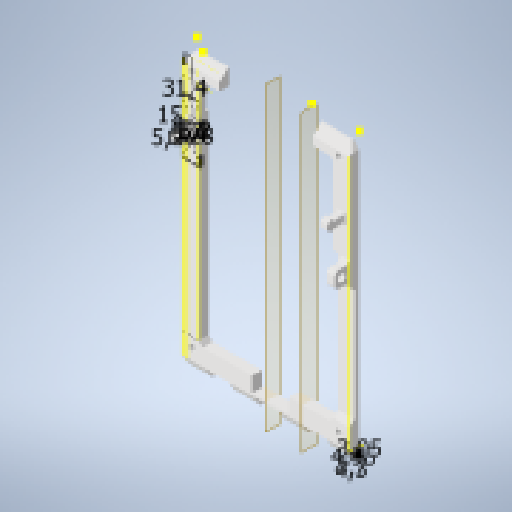
# Autodesk Inventor part: cap
Saved by Autodesk Inventor 2025 (Build 290162000, 162)
## iProperties
Created: 2026-10-31
Part Number: cap
Material: Типовые
Document SubType Name: Modeling
Designer: Leva
Density: 1 g/cm^3
Appearance: По умолчанию
Author: Leva
Autodesk Inventor part; units mm, degrees
ref_plane "YZ Plane" through (0, 0, 0) normal (1, 0, 0) x (0, 1, 0)
ref_plane "XZ Plane" through (0, 0, 0) normal (0, 1, 0) x (-1, 0, 0)
ref_plane "XY Plane" through (0, 0, 0) normal (0, 0, 1) x (1, 0, 0)
sketch "Эскиз1" plane through (0, 0, 0) normal (0, 0, 1) x (1, 0, 0)
  line L0 (72.7181, -132.5726) -> (72.7181, -8.0726) projected
  line L1 (72.7181, -8.0726) -> (69.7181, -5.0726) projected
  line L2 (69.7181, -5.0726) -> (-7.2819, -5.0726) projected
  line L3 (-7.2819, -5.0726) -> (-10.2819, -8.0726) projected
  line L4 (-10.2819, -8.0726) -> (-10.2819, -132.5726) projected
  line L5 (-10.2819, -132.5726) -> (-7.2819, -135.5726) projected
  line L6 (-7.2819, -135.5726) -> (69.7181, -135.5726) projected
  line L7 (69.7181, -135.5726) -> (72.7181, -132.5726) projected
  circle A0 centre (37.8631, -131.3876) radius 0.325 projected
  circle A1 centre (37.8631, -132.6576) radius 0.325 projected
  circle A2 centre (67.7181, -130.5726) radius 1.35 projected
  circle A3 centre (54.6891, -79.8326) radius 1.55 projected
  circle A4 centre (36.5931, -132.6576) radius 0.325 projected
  circle A5 centre (35.3231, -132.6576) radius 0.325 projected
  line L8 (17.4681, -90.7666) -> (44.9681, -90.7666) projected
  arc A6 (11.5241, -84.8226) -> (17.4681, -90.7666) centre (17.4683, -84.8225) ccw projected
  line L9 (11.5241, -57.3226) -> (11.5241, -84.8226) projected
  arc A7 (17.4681, -51.3786) -> (11.5241, -57.3226) centre (17.4683, -57.3227) ccw projected
  line L10 (44.9681, -51.3786) -> (17.4681, -51.3786) projected
  arc A8 (50.9121, -57.3226) -> (44.9681, -51.3786) centre (44.968, -57.3227) ccw projected
  line L11 (50.9121, -84.8226) -> (50.9121, -57.3226) projected
  arc A9 (44.9681, -90.7666) -> (50.9121, -84.8226) centre (44.968, -84.8225) ccw projected
  circle A10 centre (35.3231, -131.3876) radius 0.325 projected
  circle A11 centre (36.5931, -131.3876) radius 0.325 projected
  circle A12 centre (60.4681, -32.7976) radius 0.45 projected
  circle A13 centre (58.4681, -32.7976) radius 0.45 projected
  circle A14 centre (67.7181, -11.5726) radius 1.35 projected
  circle A15 centre (58.4681, -28.2976) radius 0.45 projected
  circle A16 centre (60.4681, -28.2976) radius 0.45 projected
  circle A17 centre (56.4361, -32.7976) radius 0.45 projected
  circle A18 centre (50.9731, -42.2126) radius 1.1 projected
  circle A19 centre (56.4681, -28.2976) radius 0.45 projected
  line L12 (48.1131, -37.9766) -> (14.3131, -37.9766) projected
  line L13 (14.3131, -37.9766) -> (14.3131, -7.4766) projected
  line L14 (14.3131, -7.4766) -> (48.1131, -7.4766) projected
  line L15 (48.1131, -7.4766) -> (48.1131, -37.9766) projected
  circle A20 centre (50.9731, -10.1686) radius 1.1 projected
  circle A21 centre (34.0531, -132.6576) radius 0.325 projected
  circle A22 centre (32.7831, -132.6576) radius 0.325 projected
  circle A23 centre (34.0531, -131.3876) radius 0.325 projected
  circle A24 centre (32.7831, -131.3876) radius 0.325 projected
  circle A25 centre (31.5131, -132.6576) radius 0.325 projected
  circle A26 centre (30.2431, -132.6576) radius 0.325 projected
  circle A27 centre (31.5131, -131.3876) radius 0.325 projected
  circle A28 centre (28.9731, -132.6576) radius 0.325 projected
  circle A29 centre (-5.2819, -130.5726) radius 1.35 projected
  circle A30 centre (30.2431, -131.3876) radius 0.325 projected
  circle A31 centre (28.9731, -131.3876) radius 0.325 projected
  circle A32 centre (34.2431, -122.5726) radius 1.1 projected
  circle A33 centre (34.2431, -97.5726) radius 1.1 projected
  circle A34 centre (31.2891, -47.9156) radius 1.55 projected
  circle A35 centre (11.2431, -96.7726) radius 1.1 projected
  circle A36 centre (7.8891, -79.8326) radius 1.55 projected
  circle A37 centre (11.4731, -42.2126) radius 1.1 projected
  circle A38 centre (-5.2819, -11.5726) radius 1.35 projected
  circle A39 centre (11.4731, -10.1686) radius 1.1 projected
  line L16 (-0.2819, -13.0726) -> (62.7181, -13.0726)
  line L17 (64.7181, -15.0726) -> (64.7181, -125.5726)
  line L18 (62.7181, -127.5726) -> (-0.2819, -127.5726)
  line L19 (-2.2819, -125.5726) -> (-2.2819, -15.0726)
  circle A40 centre (-5.2819, -11.5726) radius 1.8
  circle A41 centre (67.7181, -11.5726) radius 1.8
  circle A42 centre (67.7181, -130.5726) radius 1.8
  circle A43 centre (-5.2819, -130.5726) radius 1.8
  line L20 (-0.2819, -127.5726) -> (-2.2819, -125.5726)
  line L21 (-0.2819, -13.0726) -> (-2.2819, -15.0726)
  line L22 (62.7181, -13.0726) -> (64.7181, -15.0726)
  line L23 (64.7181, -125.5726) -> (62.7181, -127.5726)
  line L24 (-7.2819, -135.5726) -> (69.7181, -135.5726)
  line L25 (69.7181, -135.5726) -> (69.7181, -136.1726)
  line L26 (69.7181, -136.1726) -> (-7.2819, -136.1726)
  line L27 (-7.2819, -136.1726) -> (-7.2819, -135.5726)
  line L28 (-10.2819, -132.5726) -> (-7.2819, -132.5726)
  line L29 (-7.2819, -132.5726) -> (-7.2819, -136.1726)
  line L30 (-7.2819, -136.1726) -> (-10.2819, -136.1726)
  line L31 (-10.2819, -136.1726) -> (-10.2819, -132.5726)
  line L32 (72.7181, -132.5726) -> (69.7181, -132.5726)
  line L33 (69.7181, -132.5726) -> (69.7181, -136.1726)
  line L34 (69.7181, -136.1726) -> (72.7181, -136.1726)
  line L35 (72.7181, -136.1726) -> (72.7181, -132.5726)
  point P0 (0, 0)
  point P1 (-2.2819, -13.0726)
  point P2 (64.7181, -13.0726)
  point P3 (64.7181, -127.5726)
  point P4 (-2.2819, -127.5726)
  point P5 (69.7181, -135.5726)
  point P6 (69.7181, -135.5726)
  dimension "d0" = 8
  dimension "d1" = 3.6
  dimension "d2" = 3.6
  dimension "d3" = 3.6
  dimension "d4" = 3.6
  dimension "d5" = 2
  dimension "d6" = 2
  dimension "d7" = 2
  dimension "d8" = 2
  dimension "d9" = 2
  dimension "d10" = 2
  dimension "d11" = 2
  dimension "d12" = 2
  dimension "d35" = 77
  dimension "d36" = 0.6
  constraints: 40 end point, 8 point on line, 6 parallel, 4 centre point, 4 coincident, 3 horizontal, 3 perpendicular, 3 other
  measures "d0" distance between parallel lines of L2 L16
  measures "d1" diameter of A40
  measures "d2" diameter of A41
  measures "d3" diameter of A42
  measures "d4" diameter of A43
  measures "d5" distance of L18.end point (-2.282, -127.573)
  measures "d6" distance of L19.start point (-2.282, -127.573)
  measures "d7" distance of L16.start point (-2.282, -13.073)
  measures "d8" distance of L19.end point (-2.282, -13.073)
  measures "d9" distance of L16.end point (64.718, -13.073)
  measures "d10" distance of L17.start point (64.718, -13.073)
  measures "d11" distance of L17.end point (64.718, -127.573)
  measures "d12" distance of L18.start point (64.718, -127.573)
  measures "d35" distance of L25.end L26.end
  measures "d36" distance of L24.end L25.end
extrude "Выдавливание1" add sketch "Эскиз1" along normal blind 5 contours L32 L33 L6 L29 L28 L4 L3 L2 L1 L0 | L35 L34 L25 L7 | L7 L33 L32 | L25 L26 L27 L6 | L27 L30 L31 L5 | L5 L28 L29 | A0 | A1 | A4 | A5 | A10 | A11 | L16 L13 L14 L15 | A20 | A21 | A22 | A23 | A24 | A25 | A26 | A27 | A28 | A30 | A31 | A39
chamfer "Фаска1" distance 4 angle 45 1 edges at (31.2181, -5.0726, 5)
sketch "Эскиз2" plane through (0, 0, 5) normal (0, 0, 1) x (1, 0, 0)
  line L0 (53.4875, -42.7558) -> (53.4778, -9.7558) construction
  line L1 (8.9682, -9.7558) -> (8.9778, -42.7558) construction
  line L2 (41.6482, -134.5726) -> (41.6482, -129.4726) construction
  line L3 (25.1882, -129.4726) -> (25.1882, -134.5726) construction
  line L4 (41.6482, -134.5726) -> (42.6482, -134.5726) construction
  line L5 (42.6482, -134.5726) -> (42.6482, -135.5726) construction
  line L6 (42.6482, -135.5726) -> (41.6482, -135.5726) construction
  line L7 (41.6482, -135.5726) -> (41.6482, -134.5726) construction
  line L8 (-0.2819, -13.0726) -> (62.7181, -13.0726) construction
  line L9 (53.4788, -13.0726) -> (54.4788, -13.0726) construction
  line L10 (54.4788, -13.0726) -> (7.9688, -13.0726)
  line L11 (7.9688, -13.0726) -> (7.9688, -5.0726)
  line L12 (7.9688, -5.0726) -> (54.4788, -5.0726)
  line L13 (54.4788, -5.0726) -> (54.4788, -13.0726)
  line L14 (62.7181, -127.5726) -> (-0.2819, -127.5726) construction
  line L15 (42.6482, -135.5726) -> (24.1882, -135.5726)
  line L16 (24.1882, -135.5726) -> (24.1882, -127.5726)
  line L17 (24.1882, -127.5726) -> (42.6482, -127.5726)
  line L18 (42.6482, -127.5726) -> (42.6482, -135.5726)
  line L19 (42.6482, -135.5726) -> (24.1882, -135.5726)
  line L20 (24.1882, -135.5726) -> (24.1882, -134.5726)
  line L21 (24.1882, -134.5726) -> (42.6482, -134.5726)
  line L22 (42.6482, -134.5726) -> (42.6482, -135.5726)
  point P0 (0, 0)
  point P1 (42.6482, -134.5726)
  dimension "d18" = 1
  dimension "d19" = 1
  dimension "d20" = 1
  dimension "d21" = 46.51
  dimension "d22" = 8
  dimension "d23" = 18.46
  dimension "d40" = 1
  constraints: 34 end point, 8 parallel, 5 point on line, 4 horizontal, 4 perpendicular
  measures "d18" distance of L5.end L6.end
  measures "d19" distance of L4.end L5.end
  measures "d20" distance of L9.start L9.end
  measures "d21" distance of L11.end L12.end
  measures "d22" distance of L10.end L11.end
  measures "d23" distance of L16.end L17.end
  measures "d40" distance of L19.end L20.end
extrude "Выдавливание2" cut sketch "Эскиз2" against normal blind 5 contours L10 L11 L12 L13
sketch "Эскиз4" plane through (0, 0, 0) normal (0, 0, -1) x (-1, 0, 0)
  line L0 (2.2529, -21.7976) -> (2.2529, -22.6976) construction
  line L1 (2.2529, -24.2976) -> (2.2529, -25.1976) construction
  line L2 (2.2529, -26.7976) -> (2.2529, -27.6976) construction
  line L3 (4.2529, -20.9976) -> (2.2529, -20.9976)
  line L4 (2.2529, -20.9976) -> (2.2529, -28.4976)
  line L5 (2.2529, -28.4976) -> (4.2529, -28.4976)
  line L6 (4.2529, -28.4976) -> (4.2529, -20.9976)
  point P0 (0, 0)
  point P1 (2.2529, -24.7476)
  dimension "d26" = 2
  dimension "d27" = 7.5
  constraints: 8 end point, 2 midpoint, 2 parallel, 1 horizontal, 1 perpendicular
  measures "d26" distance of L5.end L4.end
  measures "d27" distance of L4.end L3.end
extrude "Выдавливание3" cut sketch "Эскиз4" against normal blind 1.6
sketch "Эскиз9" plane through (0, 0, 0) normal (0, 0, -1) x (-1, 0, 0)
  line L0 (10.2819, -8.0726) -> (10.2819, -136.1726) projected
  line L1 (10.2819, -136.1726) -> (-72.7181, -136.1726)
  line L2 (-72.7181, -136.1726) -> (-72.7181, -135.5726)
  line L3 (-72.7181, -135.5726) -> (10.2819, -135.5726)
  line L4 (10.2819, -135.5726) -> (10.2819, -136.1726)
  point P0 (0, 0)
  point P1 (10.2819, -135.5726)
  dimension "d58" = 83
  dimension "d59" = 0.6
  constraints: 8 end point, 2 parallel, 1 horizontal, 1 perpendicular
  measures "d58" distance of L2.end L3.end
  measures "d59" distance of L1.end L2.end
extrude "Выдавливание9" add sketch "Эскиз9" along normal blind 1.5
sketch "Эскиз12" plane through (72.7181, -136.1726, 5) normal (1, 0, 0) x (0, 0, -1)
  line L0 (0, 127.1) -> (0, 0) projected
  line L1 (0, 0) -> (4.35, 0) construction
  line L2 (4.35, 0) -> (4.35, -3.05) construction
  line L3 (4.35, -3.05) -> (0, -3.05) construction
  line L4 (0, -3.05) -> (0, 0) construction
  circle A0 centre (4.35, -3.05) radius 1.35
  circle A1 centre (4.35, -3.05) radius 2.15
  line L5 (0, 0) -> (2.5089, -4.1603)
  line L6 (6.5, 0) -> (0, 0) projected
  line L7 (0, 0) -> (6.5, 0)
  line L8 (6.5, 0) -> (6.5, -3.05)
  point P0 (5, 136.1726)
  dimension "d70" = 4.35
  dimension "d71" = 3.05
  dimension "d72" = 2.7
  dimension "d73" = 4.3
  constraints: 14 end point, 2 centre point, 2 coincident, 2 horizontal, 2 parallel, 2 point on circle, 2 tangent, 1 perpendicular
  measures "d70" distance of L2.end L3.end
  measures "d71" distance of L1.end L2.end
  measures "d72" diameter of A0
  measures "d73" diameter of A1
extrude "Выдавливание10" add sketch "Эскиз12" against normal blind 11.5
ref_plane "РабПлоскость6" through (31.2181, -8.0726, 4) normal (1, 0, 0) x (0, 0, -1)
ref_plane "РабПлоскость7" through (49.2181, -8.0726, 4) normal (1, 0, 0) x (0, 0, -1)
mirror "Зеркальное отражение2" about plane through (31.2181, -8.0726, 4) normal (1, 0, 0) of "Выдавливание10"
extrude "Выдавливание11" add sketch "Эскиз12" against normal blind 12 from surface at -23.5
pattern_linear "Прямоуг.массив2" count 2 spacing 24 along (-1, 0, 0) of "Выдавливание11"
sketch "Эскиз13" plane through (49.2181, -8.0726, 4) normal (1, 0, 0) x (0, 0, -1)
  point P0 (4, 8.0726)
sketch "Эскиз14" plane through (72.7181, -8.0726, 4) normal (1, 0, 0) x (0, 0, -1)
  circle A0 centre (3.35, -131.15) radius 1.35 projected
  line L0 (3.35, -131.15) -> (-4.65, -131.15) construction
  line L1 (-4.65, -131.15) -> (-4.65, -51.15) construction
  line L2 (-4.65, -51.15) -> (3.35, -51.15) construction
  line L3 (3.35, -51.15) -> (3.35, -131.15) construction
  circle A1 centre (-4.65, -51.15) radius 1.75
  line L4 (-1, -117.5) -> (-1, -7) projected
  line L5 (-8.3, -47.15) -> (-1, -47.15)
  line L6 (-1, -47.15) -> (-1, -55.15)
  line L7 (-1, -55.15) -> (-8.3, -55.15)
  line L8 (-8.3, -55.15) -> (-8.3, -47.15)
  line L9 (-8.3, -47.15) -> (-1, -55.15) construction
  line L10 (-1, -47.15) -> (-8.3, -55.15) construction
  point P0 (4, 8.0726)
  point P1 (-1, -47.15)
  dimension "d82" = 8
  dimension "d83" = 80
  dimension "d84" = 3.5
  dimension "d85" = 8
  constraints: 20 end point, 4 parallel, 2 horizontal, 2 midpoint, 2 perpendicular, 1 centre point, 1 coincident, 1 point on line
  measures "d82" distance of L1.end L2.end
  measures "d83" distance of L0.end L1.end
  measures "d84" diameter of A1
  measures "d85" distance of L5.end L6.end
extrude "Выдавливание12" add sketch "Эскиз14" against normal blind 3.9 contours L7 L8 L5 L4
fillet "Сопряжение1" radius 2 2 edges at (70.7681, -63.2226, 12.3) (70.7681, -55.2226, 12.3)
sketch "Эскиз17" plane through (0, 0, 5) normal (0, 0, 1) x (1, 0, 0)
  line L0 (-6.3819, 7.1) -> (-10.2819, 7.1) projected
  line L1 (-10.2819, 7.1) -> (-10.2819, 5.1) construction
  line L2 (-10.2819, -8.0726) -> (-10.2819, -135.5726) projected
  line L3 (72.7181, -63.2226) -> (68.8181, -63.2226) projected
  line L4 (72.7181, -63.2226) -> (72.7181, -65.2226) construction
  line L5 (72.7181, -135.5726) -> (72.7181, -8.0726) projected
  line L6 (-0.2819, -127.5726) -> (-2.2819, -125.5726) projected
  line L7 (-10.2819, 5.1) -> (-2.2819, 5.1)
  line L8 (-2.2819, 5.1) -> (-2.2819, -125.5726)
  line L9 (-2.2819, -125.5726) -> (-10.2819, -125.5726)
  line L10 (-10.2819, -125.5726) -> (-10.2819, 5.1)
  line L11 (64.7181, -15.0726) -> (64.7181, -125.5726) projected
  line L12 (72.7181, -65.2226) -> (64.7181, -65.2226)
  line L13 (64.7181, -65.2226) -> (64.7181, -125.5726)
  line L14 (64.7181, -125.5726) -> (72.7181, -125.5726)
  line L15 (72.7181, -125.5726) -> (72.7181, -65.2226)
  line L16 (-6.3819, 7.1) -> (-6.3819, 5.1) construction
  line L17 (-6.3819, 5.1) -> (-2.2819, 5.1)
  line L18 (-2.2819, 5.1) -> (-2.2819, 15.1)
  line L19 (-2.2819, 15.1) -> (-6.3819, 15.1)
  line L20 (-6.3819, 15.1) -> (-6.3819, 5.1)
  line L21 (68.8181, -63.2226) -> (68.8181, -61.2226) construction
  line L22 (68.8181, -63.2226) -> (68.8181, -65.2226) construction
  line L23 (68.8181, -65.2226) -> (64.7181, -65.2226)
  line L24 (64.7181, -65.2226) -> (64.7181, -53.2226)
  line L25 (64.7181, -53.2226) -> (68.8181, -53.2226)
  line L26 (68.8181, -53.2226) -> (68.8181, -65.2226)
  point P0 (0, 0)
  point P1 (72.7181, -125.5726)
  point P2 (-10.2819, -125.5726)
  point P3 (64.7181, -53.2226)
  dimension "d96" = 2
  dimension "d97" = 2
  dimension "d106" = 4.1
  dimension "d107" = 10
  dimension "d108" = 4.1
  dimension "d109" = 12
  constraints: 40 end point, 8 parallel, 6 perpendicular, 4 horizontal, 4 point on line
  measures "d96" distance of L0.end L1.end
  measures "d97" distance of L3.start L4.end
  measures "d106" distance of L19.end L18.end
  measures "d107" distance of L18.end L17.end
  measures "d108" distance of L24.end L25.end
  measures "d109" distance of L23.end L24.end
extrude "Выдавливание15" cut sketch "Эскиз17" against normal blind 2.5 contours L26 L12 L11 L25 | L5 L14 L11 L12
chamfer "Фаска4" distance 2 angle 45 2 edges at (70.7681, -63.2226, 5) (70.7681, -55.2226, 5)
chamfer "Фаска5" distance 2.5 angle 45 3 edges at (70.7681, -65.2226, 2.5) (68.7181, -125.5726, 2.5) (66.7681, -53.2226, 2.5)
sketch "Эскиз18" plane through (0, 0, 5) normal (0, 0, 1) x (1, 0, 0)
  line L0 (-2.2819, -15.0726) -> (-10.2819, -15.0726) construction
  line L1 (-10.2819, -8.0726) -> (-10.2819, -135.5726) projected
  line L2 (-2.2819, -125.5726) -> (-2.2819, -15.0726) projected
  line L3 (-2.2819, -125.5726) -> (-10.2819, -125.5726) construction
  line L4 (-6.2819, -15.0726) -> (-6.2819, -5.0726) construction
  line L5 (7.9688, -5.0726) -> (-7.2819, -5.0726) construction
  line L6 (-6.2819, -5.0726) -> (-6.2819, -36.4726) construction
  line L7 (-6.2819, -28.9726) -> (-6.2819, -43.9726) construction
  line L8 (-7.9819, -34.8726) -> (-4.5819, -34.8726)
  line L9 (-4.5819, -34.8726) -> (-4.5819, -38.0726)
  line L10 (-4.5819, -38.0726) -> (-7.9819, -38.0726)
  line L11 (-7.9819, -38.0726) -> (-7.9819, -34.8726)
  line L12 (-7.9819, -34.8726) -> (-4.5819, -38.0726) construction
  line L13 (-4.5819, -34.8726) -> (-7.9819, -38.0726) construction
  line L14 (-7.9819, -33.8726) -> (-4.5819, -33.8726)
  line L15 (-4.5819, -33.8726) -> (-4.5819, -39.0726)
  line L16 (-4.5819, -39.0726) -> (-7.9819, -39.0726)
  line L17 (-7.9819, -39.0726) -> (-7.9819, -33.8726)
  line L18 (-7.9819, -33.8726) -> (-4.5819, -39.0726) construction
  line L19 (-4.5819, -33.8726) -> (-7.9819, -39.0726) construction
  line L20 (-2.2819, -28.4976) -> (-2.2819, -20.9976) projected
  line L21 (-10.2819, -50.4726) -> (-2.2819, -50.4726)
  line L22 (-2.2819, -50.4726) -> (-2.2819, -22.4726)
  line L23 (-2.2819, -22.4726) -> (-10.2819, -22.4726)
  line L24 (-10.2819, -22.4726) -> (-10.2819, -50.4726)
  line L25 (-10.2819, -50.4726) -> (-2.2819, -22.4726) construction
  line L26 (-2.2819, -50.4726) -> (-10.2819, -22.4726) construction
  point P0 (0, 0)
  dimension "d110" = 31.4
  dimension "d111" = 15
  dimension "d112" = 3.4
  dimension "d113" = 3.2
  dimension "d114" = 3.4
  dimension "d115" = 5.2
  dimension "d116" = 28
  constraints: 46 end point, 8 midpoint, 7 parallel, 5 horizontal, 4 point on line, 3 perpendicular, 1 vertical
  measures "d110" distance of L6.end L4.end
  measures "d111" distance of L7.start L7.end
  measures "d112" distance of L9.end L10.end
  measures "d113" distance of L8.end L9.end
  measures "d114" distance of L15.end L16.end
  measures "d115" distance of L14.end L15.end
  measures "d116" distance of L22.end L21.end
extrude "Выдавливание19" add sketch "Эскиз18" along normal blind 5.93 contours L8 L9 L10 L11
extrude "Выдавливание20" add sketch "Эскиз18" along normal blind 2.6 from surface at 5.93 contours L17 L14 L15 L8 | L8 L9 L10 L11 | L10 L15 L16 L17
chamfer "Фаска8" distance 1.4 angle 45 2 edges at (-6.2819, -39.0726, 13.53) (-6.2819, -33.8726, 13.53)
chamfer "Фаска9" distance 0.8 angle 45 4 edges at (-7.9819, -36.4726, 5) (-6.2819, -38.0726, 5) (-4.5819, -36.4726, 5) (-6.2819, -34.8726, 5)
mirror "Зеркальное отражение4" about plane through (31.2181, -8.0726, 4) normal (1, 0, 0) of "Выдавливание19", "Выдавливание20", "Фаска8", "Фаска9"
sketch "Эскиз20" plane through (-7.9819, -39.0726, 10.93) normal (-1, 0, 0) x (0, 0, 1)
  line L0 (-5.13, 1) -> (-5.93, 0.2) projected
  line L1 (-5.93, 0.2) -> (-5.93, 0) construction
  line L2 (-5.93, 30) -> (-5.93, -97.1) projected
  line L3 (-5.93, 0) -> (3.07, 0)
  line L4 (3.07, 0) -> (3.07, 5.2)
  line L5 (3.07, 5.2) -> (-5.93, 5.2)
  line L6 (-5.93, 5.2) -> (-5.93, 0)
  point P0 (-10.93, 39.0726)
  point P1 (-5.93, 5.2)
  dimension "d139" = 0.2
  dimension "d140" = 9
  dimension "d141" = 5.2
  constraints: 10 end point, 2 parallel, 1 horizontal, 1 perpendicular, 1 point on line
  measures "d139" distance of L0.end L1.end
  measures "d140" distance of L5.end L4.end
  measures "d141" distance of L4.end L3.end
sketch "Эскиз21" plane through (0, 0, 5) normal (0, 0, 1) x (1, 0, 0)
  line L0 (25.1882, -129.4726) -> (25.1882, -134.5726) projected
  line L1 (25.1882, -134.5726) -> (41.6482, -134.5726) projected
  line L2 (41.6482, -134.5726) -> (41.6482, -129.4726) projected
  line L3 (25.1882, -129.4726) -> (24.1882, -129.4726) construction
  line L4 (24.1882, -129.4726) -> (24.1882, -127.5726) construction
  line L5 (24.1882, -127.5726) -> (25.1882, -127.5726) construction
  line L6 (25.1882, -127.5726) -> (25.1882, -129.4726) construction
  line L7 (24.1882, -127.5726) -> (24.1882, -134.9726)
  line L8 (13.2181, -136.1726) -> (25.2181, -136.1726) projected
  line L9 (24.1882, -134.9726) -> (42.6482, -134.9726)
  line L10 (42.6482, -134.9726) -> (42.6482, -127.5726)
  line L11 (24.1882, -127.5726) -> (42.6482, -127.5726)
  point P0 (0, 0)
  dimension "d144" = 1
  dimension "d145" = 1.9
  dimension "d146" = 7.4
  dimension "d147" = 18.46
  constraints: 16 end point, 3 parallel, 3 perpendicular, 2 horizontal
  measures "d144" distance of L4.end L5.end
  measures "d145" distance of L3.end L4.end
  measures "d146" distance of L4.end L7.end
  measures "d147" distance of L7.end L9.end
extrude "Выдавливание22" cut sketch "Эскиз21" against normal blind 10
equation "\"d6\" = d5"
equation "\"d7\" = d5"
equation "\"d8\" = d7"
equation "\"d9\" = d5"
equation "\"d10\" = d9"
equation "\"d11\" = d5"
equation "\"d12\" = d11"
